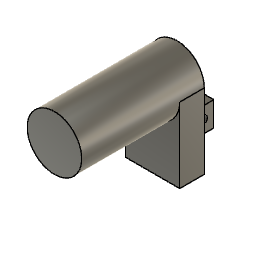
MotorAssemblyCombinedLinearActuator v9 (Autodesk Fusion 360 archive; units mm, degrees)
design "Linear Actuator"
Autodesk Fusion 360 part; units mm, degrees
sketch "Sketch1" plane through (0, 0, 0) normal (0, 0, 1) x (1, 0, 0)
sketch "Sketch2" plane through (0, 0, 0) normal (1, 0, 0) x (0, 1, 0)
  line L0 (36, -20) -> (-36, -20)
  line L1 (-36, -20) -> (-36, 20)
  line L2 (-36, 20) -> (36, 20)
  line L3 (36, 20) -> (36, -20)
  line L4 (36, -20) -> (-36, 20) construction
  line L5 (-36, -20) -> (36, 20) construction
  dimension "d1" = 72
  dimension "d2" = 40
  constraint horizontal L0
  constraint perpendicular L0 L1
  constraint parallel L0 L2
  constraint parallel L1 L3
  constraint coincident L4 origin
  constraint coincident L5 origin
  measures "d1" distance of L1.end L2.end
  measures "d2" distance of L0.end L1.end
sketch "Sketch3" plane through (0, 0, 0) normal (0, 1, 0) x (1, 0, 0)
  circle A0 centre (0, 0) radius 20
  dimension "d3" = 40
  constraint coincident A0.centre origin
  measures "d3" diameter of A0
extrude "Extrude1" add sketch "Sketch3" along normal mid plane 72
sketch "Sketch4" plane through (0, 0, 0) normal (0, 1, 0) x (1, 0, 0)
sketch "Sketch5" plane through (0, 36, 0) normal (0, 1, 0) x (-1, 0, 0)
  circle A0 centre (0, 0) radius 20
  circle A1 centre (0, 0) radius 20
  line L0 (0, 20) -> (0, -55) construction
  line L1 (20, 0) -> (20, -55)
  line L2 (20, -55) -> (-20, -55)
  line L3 (-20, -55) -> (-20, 0)
  line L4 (0, -55) -> (0, -31) construction
  line L5 (9, -40) -> (-9, -40)
  line L6 (-9, -40) -> (-9, -22)
  line L7 (-9, -22) -> (9, -22)
  line L8 (9, -22) -> (9, -40)
  line L9 (9, -40) -> (-9, -22) construction
  line L10 (-9, -40) -> (9, -22) construction
  line L11 (20, -19.9504) -> (-20, -19.9504)
  line L12 (-20, -19.9504) -> (-20, -49.9504)
  line L13 (-20, -49.9504) -> (20, -49.9504)
  line L14 (20, -49.9504) -> (20, -19.9504)
  point P0 (0, -31)
  dimension "d6" = 75
  dimension "d11" = 24
  dimension "d12" = 18
  dimension "d21" = 30
  constraint concentric A0 A1
  constraint coincident A1 L0.start
  constraint vertical L0
  constraint vertical L1
  constraint horizontal L2
  constraint vertical L3
  constraint coincident A0 L1.start
  constraint coincident A0 L3.end
  constraint parallel L0 L4
  constraint horizontal L5
  constraint perpendicular L5 L6
  constraint parallel L5 L7
  constraint parallel L6 L8
  constraint coincident L9 P0
  constraint coincident L10 P0
  constraint coincident P0 L4.end
  constraint horizontal L11
  constraint vertical L12
  constraint horizontal L13
  constraint vertical L14
  constraint coincident L1 L11.start
  measures "d6" distance of L0.start L0.end
  measures "d11" distance of L0.end P0
  measures "d12" distance of L6.end L7.end
  measures "d21" distance of L11.start L13.end
extrude "Extrude2" add sketch "Sketch5" along normal blind 18 contours A0 A1 L11 | A0 A1 L1 L11 | A0 A1 L3 L11 | A0 A1 L1 L3 L11 L12 L13 L14 | A0 A1 L11 | L1 L2 L3 L13 | L5 L6 L7 L8
extrude "Extrude4" add sketch "Sketch5" along normal blind 36 contours L5 L6 L7 L8
sketch "Sketch6" plane through (0, 0, 0) normal (1, 0, 0) x (0, 1, 0)
  line L0 (54, -22) -> (72, -40) construction
  line L1 (72, -40) -> (72, -22) construction
  line L2 (72, -22) -> (54, -40) construction
  line L3 (54, -40) -> (63, -31) construction
  line L4 (54, -31) -> (64, -31) construction
  circle A0 centre (64, -31) radius 3.25
  dimension "d17" = 10
  dimension "d18" = 6.5
  constraint vertical L1
  constraint perpendicular L0 L2
  constraint midpoint L0 L3.end
  constraint perpendicular L0 L3
  constraint horizontal L4
  constraint coincident L4.end A0.centre
  measures "d17" distance of L4.start L4.end
  measures "d18" diameter of A0
extrude "Extrude5" cut sketch "Sketch6" along normal mid plane 64
extrude "Extrude6" [suppressed]
extrude "Extrude3" [suppressed]

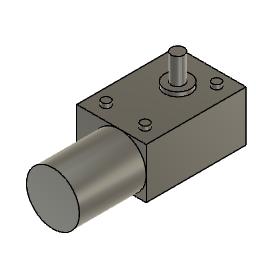
design "Motor-JGY"
Autodesk Fusion 360 part; units mm, degrees
sketch "Mounting" plane through (0, 0, 0) normal (0, 0, 1) x (1, 0, 0)
  line L0 (9, -16.5) -> (-9, -16.5) construction
  line L1 (-9, -16.5) -> (-9, 16.5) construction
  line L2 (-9, 16.5) -> (9, 16.5) construction
  line L3 (9, 16.5) -> (9, -16.5) construction
  line L4 (9, -16.5) -> (-9, 16.5) construction
  line L5 (-9, -16.5) -> (9, 16.5) construction
  circle A0 centre (-9, 16.5) radius 2
  circle A1 centre (9, 16.5) radius 2
  circle A2 centre (9, -16.5) radius 2
  circle A3 centre (-9, -16.5) radius 2
  line L6 (16, -23) -> (-16, -23)
  line L7 (-16, -23) -> (-16, 23)
  line L8 (-16, 23) -> (16, 23)
  line L9 (16, 23) -> (16, -23)
  line L10 (16, -23) -> (-16, 23) construction
  line L11 (-16, -23) -> (16, 23) construction
  line L12 (-9, 16.5) -> (-9, 7.5) construction
  line L13 (-9, 7.5) -> (0, 7.5) construction
  circle A4 centre (0, 7.5) radius 6
  circle A5 centre (0, 7.5) radius 3
  dimension "d1" = 18
  dimension "d2" = 33
  dimension "d3" = 4
  dimension "d4" = 4
  dimension "d5" = 4
  dimension "d6" = 4
  dimension "d7" = 32
  dimension "d8" = 46
  dimension "d9" = 9
  dimension "d10" = 9
  dimension "d11" = 12
  dimension "d12" = 6
  constraint horizontal L0
  constraint perpendicular L0 L1
  constraint parallel L0 L2
  constraint parallel L1 L3
  constraint coincident L4 origin
  constraint coincident L5 origin
  constraint coincident L1.end L2.start
  constraint coincident L2.end L3.start
  constraint coincident L0.start L3.end
  constraint coincident L0.end L1.start
  constraint horizontal L6
  constraint perpendicular L6 L7
  constraint parallel L6 L8
  constraint parallel L7 L9
  constraint coincident L10 origin
  constraint coincident L11 origin
  constraint parallel L1 L12
  constraint perpendicular L12 L13
  constraint coincident L13.end A4.centre
  constraint concentric A4 A5
  measures "d1" distance of L1.end L2.end
  measures "d2" distance of L0.end L1.end
  measures "d3" diameter of A0
  measures "d4" diameter of A1
  measures "d5" diameter of A2
  measures "d6" diameter of A3
  measures "d7" distance of L7.end L8.end
  measures "d8" distance of L6.end L7.end
  measures "d9" distance of L1.end L12.end
  measures "d10" distance of L12.end L13.end
  measures "d11" diameter of A4
  measures "d12" diameter of A5
extrude "Extrude1" add sketch "Mounting" along normal blind 14 contours A5 makes body 1
extrude "Extrude2" add sketch "Mounting" along normal blind 2 contours A0 | A1 | A2 | A3 | A4 bodies 1 makes body 2 at (10.9975, -16.5997, 1.3333) makes body 3 at (10.9975, 16.4003, 1.3333) makes body 4 at (-7.0025, -16.5997, 1.3333) makes body 5 at (-7.0025, 16.4003, 1.3333)
extrude "Extrude3" add sketch "Mounting" against normal blind 25.2 separate body contours L6 L7 L8 L9 makes body 6
extrude "Extrude6" cut sketch "Mounting" against normal blind 29 contours L6 L7 L8 L9 bodies 6
extrude "Extrude7" add sketch "Mounting" against normal blind 23.2 contours L6 L7 L8 L9 bodies 6 1 2 3 4 5
sketch "Motor" plane through (0, -23, 0) normal (0, -1, 0) x (1, 0, 0)
  line L0 (16, 0) -> (-16, 0)
  line L1 (-16, 0) -> (-16, -23.2)
  line L2 (-16, -23.2) -> (16, -23.2)
  line L3 (16, -23.2) -> (16, 0)
  line L4 (-16, 0) -> (16, -23.2) construction
  line L5 (-16, -23.2) -> (16, 0) construction
  line L6 (16, 0) -> (-16, 0) construction
  circle A0 centre (3.8, -12.2) radius 12.2
  dimension "d29" = 12.2
  constraint coincident L0.end L1.start
  constraint coincident L2.end L3.start
  constraint coincident L1.end L2.start
  constraint coincident L0.start L3.end
  constraint tangent L3 A0
  constraint tangent L6 A0
  measures "d29" radius of A0
extrude "Extrude8" add sketch "Motor" along normal blind 30.8 separate body contours L2 A0 picked at (8.1727, -6.557) makes body 7
extrude "Extrude9" add sketch "Mounting" against normal blind 23.2 contours A0 | A1 | A2 | A3 | L6 L7 L8 L9 | A4 | A5 bodies 6 7
extrude "Extrude11" add sketch "Motor" along normal blind 30.8 contours L2 A0 picked at (4.9947, -23.4206) bodies 6
ref_plane "WorkPlane1" through (0, 0, 2) normal (0, 0, 1) x (1, 0, 0)
sketch "Sketch4" plane through (0, 0, 2) normal (0, 0, 1) x (1, 0, 0)
  line L0 (-20, 25) -> (20, 25)
  line L1 (20, 25) -> (20, -23)
  line L2 (20, -23) -> (-20, -23)
  line L3 (-20, -23) -> (-20, 25)
  circle A0 centre (0, 7.5) radius 3.25
  dimension "d39" = 6.5
  constraint horizontal L0
  constraint vertical L1
  constraint horizontal L2
  constraint vertical L3
  measures "d39" diameter of A0
extrude "Extrude10" [suppressed]
extrude "Extrude5" [suppressed]
extrude "Extrude4" [suppressed]

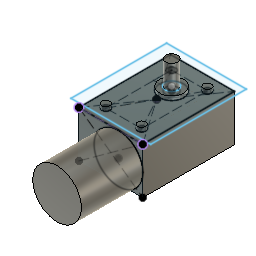
design "Motor-JGY"
Autodesk Fusion 360 part; units mm, degrees
sketch "Mounting" plane through (0, 0, 0) normal (0, 0, 1) x (1, 0, 0)
  line L0 (9, -16.5) -> (-9, -16.5) construction
  line L1 (-9, -16.5) -> (-9, 16.5) construction
  line L2 (-9, 16.5) -> (9, 16.5) construction
  line L3 (9, 16.5) -> (9, -16.5) construction
  line L4 (9, -16.5) -> (-9, 16.5) construction
  line L5 (-9, -16.5) -> (9, 16.5) construction
  circle A0 centre (-9, 16.5) radius 2
  circle A1 centre (9, 16.5) radius 2
  circle A2 centre (9, -16.5) radius 2
  circle A3 centre (-9, -16.5) radius 2
  line L6 (16, -23) -> (-16, -23)
  line L7 (-16, -23) -> (-16, 23)
  line L8 (-16, 23) -> (16, 23)
  line L9 (16, 23) -> (16, -23)
  line L10 (16, -23) -> (-16, 23) construction
  line L11 (-16, -23) -> (16, 23) construction
  line L12 (-9, 16.5) -> (-9, 7.5) construction
  line L13 (-9, 7.5) -> (0, 7.5) construction
  circle A4 centre (0, 7.5) radius 6
  circle A5 centre (0, 7.5) radius 3
  dimension "d1" = 18
  dimension "d2" = 33
  dimension "d3" = 4
  dimension "d4" = 4
  dimension "d5" = 4
  dimension "d6" = 4
  dimension "d7" = 32
  dimension "d8" = 46
  dimension "d9" = 9
  dimension "d10" = 9
  dimension "d11" = 12
  dimension "d12" = 6
  constraint horizontal L0
  constraint perpendicular L0 L1
  constraint parallel L0 L2
  constraint parallel L1 L3
  constraint coincident L4 origin
  constraint coincident L5 origin
  constraint coincident L1.end L2.start
  constraint coincident L2.end L3.start
  constraint coincident L0.start L3.end
  constraint coincident L0.end L1.start
  constraint horizontal L6
  constraint perpendicular L6 L7
  constraint parallel L6 L8
  constraint parallel L7 L9
  constraint coincident L10 origin
  constraint coincident L11 origin
  constraint parallel L1 L12
  constraint perpendicular L12 L13
  constraint coincident L13.end A4.centre
  constraint concentric A4 A5
  measures "d1" distance of L1.end L2.end
  measures "d2" distance of L0.end L1.end
  measures "d3" diameter of A0
  measures "d4" diameter of A1
  measures "d5" diameter of A2
  measures "d6" diameter of A3
  measures "d7" distance of L7.end L8.end
  measures "d8" distance of L6.end L7.end
  measures "d9" distance of L1.end L12.end
  measures "d10" distance of L12.end L13.end
  measures "d11" diameter of A4
  measures "d12" diameter of A5
extrude "Extrude1" add sketch "Mounting" along normal blind 14 contours A5 makes body 1
extrude "Extrude2" add sketch "Mounting" along normal blind 2 contours A0 | A1 | A2 | A3 | A4 bodies 1 makes body 2 at (10.9975, -16.5997, 1.3333) makes body 3 at (10.9975, 16.4003, 1.3333) makes body 4 at (-7.0025, -16.5997, 1.3333) makes body 5 at (-7.0025, 16.4003, 1.3333)
extrude "Extrude3" add sketch "Mounting" against normal blind 25.2 separate body contours L6 L7 L8 L9 makes body 6
extrude "Extrude6" cut sketch "Mounting" against normal blind 29 contours L6 L7 L8 L9 bodies 6
extrude "Extrude7" add sketch "Mounting" against normal blind 23.2 contours L6 L7 L8 L9 bodies 6 1 2 3 4 5
sketch "Motor" plane through (0, -23, 0) normal (0, -1, 0) x (1, 0, 0)
  line L0 (16, 0) -> (-16, 0)
  line L1 (-16, 0) -> (-16, -23.2)
  line L2 (-16, -23.2) -> (16, -23.2)
  line L3 (16, -23.2) -> (16, 0)
  line L4 (-16, 0) -> (16, -23.2) construction
  line L5 (-16, -23.2) -> (16, 0) construction
  line L6 (16, 0) -> (-16, 0) construction
  circle A0 centre (3.8, -12.2) radius 12.2
  dimension "d29" = 12.2
  constraint coincident L0.end L1.start
  constraint coincident L2.end L3.start
  constraint coincident L1.end L2.start
  constraint coincident L0.start L3.end
  constraint tangent L3 A0
  constraint tangent L6 A0
  measures "d29" radius of A0
extrude "Extrude8" add sketch "Motor" along normal blind 30.8 separate body contours L2 A0 picked at (8.1727, -6.557) makes body 7
extrude "Extrude9" add sketch "Mounting" against normal blind 23.2 contours A0 | A1 | A2 | A3 | L6 L7 L8 L9 | A4 | A5 bodies 6 7
extrude "Extrude11" add sketch "Motor" along normal blind 30.8 contours L2 A0 picked at (4.9947, -23.4206) bodies 6
ref_plane "WorkPlane1" through (0, 0, 2) normal (0, 0, 1) x (1, 0, 0)
sketch "Sketch4" plane through (0, 0, 2) normal (0, 0, 1) x (1, 0, 0)
  line L0 (-20, 25) -> (20, 25)
  line L1 (20, 25) -> (20, -23)
  line L2 (20, -23) -> (-20, -23)
  line L3 (-20, -23) -> (-20, 25)
  circle A0 centre (0, 7.5) radius 3.25
  dimension "d39" = 6.5
  constraint horizontal L0
  constraint vertical L1
  constraint horizontal L2
  constraint vertical L3
  measures "d39" diameter of A0
extrude "Extrude10" [suppressed]
extrude "Extrude5" [suppressed]
extrude "Extrude4" [suppressed]
